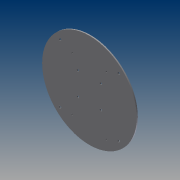
# Autodesk Inventor part: BaseTop
Saved by Autodesk Inventor 2011 SP1 (Build 150282100, 282)
## iProperties
Created: 2011-07-18
Part Number: BaseTop
Document SubType Name: Modeling
Designer: Nathan
Density: 1 g/cm^3
Author: Nathan
Autodesk Inventor part; units mm, degrees
ref_plane "YZ Plane" through (0, 0, 0) normal (1, 0, 0) x (0, 1, 0)
ref_plane "XZ Plane" through (0, 0, 0) normal (0, 1, 0) x (-1, 0, 0)
ref_plane "XY Plane" through (0, 0, 0) normal (0, 0, 1) x (1, 0, 0)
sketch "Sketch1" plane through (0, 0, 0) normal (0, 0, 1) x (1, 0, 0)
  line L0 (0, 3.1673) -> (0, -2.4908)
  line L1 (-20.5368, 0) -> (25.7294, 0)
  line L2 (0, 0) -> (-9.8402, -9.8402)
  line L3 (0, 0) -> (13.9161, 0) construction
  line L4 (0, 0) -> (-23.2805, 23.2805)
  circle A0 centre (0, 0) radius 66.675
  point P0 (-16.1645, 16.1645)
  point P1 (-41.3092, 41.3092)
  point P2 (-41.3092, -41.3092)
  point P3 (-16.1645, -16.1645)
  point P4 (16.1645, 16.1645)
  point P5 (41.3092, 41.3092)
  point P6 (41.3092, -41.3092)
  point P7 (16.1645, -16.1645)
  point P8 (24.13, -47.9739)
  point P9 (24.13, 34.5761)
  point P10 (-24.13, 33.3061)
  point P11 (-24.13, -41.6239)
  dimension "d1" = 45
  dimension "d57" = 35.56
  dimension "d58" = 22.86
  dimension "d59" = 48.26
  dimension "d60" = 48.26
  dimension "d61" = 74.93
  dimension "d62" = 82.55
  dimension "d63" = 6.35
  dimension "d64" = 1.27
  dimension "d65" = 24.13
  dimension "d66" = 133.35
  constraints: 10 end point, 6 symmetric about line, 2 horizontal, 2 perpendicular, 2 point on line, 2 vertical, 1 centre point, 1 coincident, 1 equal length
  measures "d1" angle of L3 L2
  measures "d57" distance of point (-41.309, 41.309) point (-16.164, 16.164)
  measures "d58" distance of L2.start point (-16.164, 16.164)
  measures "d59" horizontal distance of point (24.13, 34.576) point (-24.13, 33.306)
  measures "d60" horizontal distance of point (-24.13, -41.624) point (24.13, -47.974)
  measures "d61" distance of point (-24.13, -41.624) point (-24.13, 33.306)
  measures "d62" distance of point (24.13, 34.576) point (24.13, -47.974)
  measures "d63" vertical distance of point (-24.13, -41.624) point (24.13, -47.974)
  measures "d64" vertical distance of point (24.13, 34.576) point (-24.13, 33.306)
  measures "d65" distance from line of L0 point (-24.13, -41.624)
  measures "d66" diameter of A0
extrude "Extrusion1" add sketch "Sketch1" along normal blind 1.5875
hole "Hole1" at (-16.1645, 16.1645, 0) at (-41.3092, 41.3092, 0) at (-41.3092, -41.3092, 0) at (-16.1645, -16.1645, 0) at (41.3092, 41.3092, 0) at (16.1645, 16.1645, 0) at (16.1645, -16.1645, 0) at (41.3092, -41.3092, 0) direction (0, 0, 1) diameter 3.302 end through all thread size "8-32 UNC" class "2B" standard "ANSI Unified Screw Threads"
hole "Hole2" at (24.13, -47.9739, 0) at (24.13, 34.5761, 0) at (-24.13, 33.3061, 0) at (-24.13, -41.6239, 0) direction (0, 0, 1) diameter 2.159 end through all
body "Solid1"
